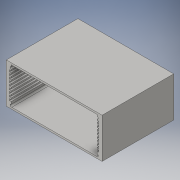
# Autodesk Inventor part: 40mm_Case
Saved by Autodesk Inventor 2016 (Build 200138000, 138)
## iProperties
Created: 2016-09-07
Part Number: 40mm_Case
Material: Generic
Document SubType Name: Modeling
Designer: jfixelle
Density: 1 g/cm^3
Appearance: Default
Author: jfixelle
Autodesk Inventor part; units mm, degrees
ref_plane "YZ Plane" through (0, 0, 0) normal (1, 0, 0) x (0, 1, 0)
ref_plane "XZ Plane" through (0, 0, 0) normal (0, 1, 0) x (-1, 0, 0)
ref_plane "XY Plane" through (0, 0, 0) normal (0, 0, 1) x (1, 0, 0)
sketch "Sketch2" plane through (0, 0, 0) normal (0, 0, 1) x (1, 0, 0)
  line L0 (-53.825, 22.5) -> (53.825, 22.5)
  line L1 (53.825, 22.5) -> (53.825, -22.5)
  line L2 (53.825, -22.5) -> (-53.825, -22.5)
  line L3 (-53.825, -22.5) -> (-53.825, 22.5)
  line L4 (-48.25, 20.5) -> (48.25, 20.5)
  line L5 (48.25, -20.5) -> (-48.25, -20.5)
  line L6 (-50.25, 19.8997) -> (-50.25, -18.4997)
  line L7 (50.25, 19.3484) -> (50.25, -18.4997)
  line L8 (48.25, 14.7) -> (50.25, 14.7)
  line L9 (-50.25, 14.7) -> (-48.25, 14.7)
  line L10 (-50.25, -15.3) -> (-48.25, -15.3)
  line L11 (48.25, -15.3) -> (50.25, -15.3)
  line L12 (49.25, 14.7) -> (49.25, -15.3) construction
  line L13 (49.25, -0.3) -> (-49.8494, -0.3) construction
  line L14 (48.25, -1.3) -> (50.25, -1.3)
  line L15 (50.25, 0.7) -> (48.25, 0.7)
  line L16 (-48.25, 0.7) -> (-50.25, 0.7)
  line L17 (-48.25, -1.3) -> (-50.25, -1.3)
  line L18 (-50.25, 2.2) -> (-48.25, 2.2)
  line L19 (48.25, 2.2) -> (50.25, 2.2)
  line L20 (-50.25, -2.8) -> (-48.25, -2.8)
  line L21 (48.25, -2.8) -> (50.25, -2.8)
  line L22 (-48.25, 4.2) -> (-50.25, 4.2)
  line L23 (48.25, 4.2) -> (50.25, 4.2)
  line L24 (50.25, -4.8) -> (48.25, -4.8)
  line L25 (-48.25, -4.8) -> (-50.25, -4.8)
  line L26 (48.25, -1.3) -> (48.25, -2.8)
  line L27 (48.25, 2.2) -> (48.25, 0.7)
  line L28 (-48.25, -2.8) -> (-48.25, -1.3)
  line L29 (-48.25, 0.7) -> (-48.25, 2.2)
  line L30 (-48.25, -6.3) -> (-50.25, -6.3)
  line L31 (48.25, -6.3) -> (50.25, -6.3)
  line L32 (48.25, -8.3) -> (50.25, -8.3)
  line L33 (-48.25, -8.3) -> (-50.25, -8.3)
  line L34 (-50.25, -9.8) -> (-48.25, -9.8)
  line L35 (48.25, -9.8) -> (50.25, -9.8)
  line L36 (50.25, -11.8) -> (48.25, -11.8)
  line L37 (-48.25, -11.8) -> (-50.25, -11.8)
  line L38 (-50.25, -13.3) -> (-48.25, -13.3)
  line L39 (48.25, -13.3) -> (50.25, -13.3)
  line L40 (50.25, 5.7) -> (48.25, 5.7)
  line L41 (-48.25, 5.7) -> (-50.25, 5.7)
  line L42 (-50.25, 7.7) -> (-48.25, 7.7)
  line L43 (48.25, 7.7) -> (50.25, 7.7)
  line L44 (50.25, 9.2) -> (48.25, 9.2)
  line L45 (-48.25, 9.2) -> (-50.25, 9.2)
  line L46 (-50.25, 11.2) -> (-48.25, 11.2)
  line L47 (48.25, 11.2) -> (50.25, 11.2)
  line L48 (50.25, 12.7) -> (48.25, 12.7)
  line L49 (-48.25, 12.7) -> (-50.25, 12.7)
  line L50 (48.25, -4.8) -> (48.25, -6.3)
  line L51 (48.25, -8.3) -> (48.25, -9.8)
  line L52 (48.25, -11.8) -> (48.25, -13.3)
  line L53 (48.25, -15.3) -> (48.25, -20.5)
  line L54 (48.25, 5.7) -> (48.25, 4.2)
  line L55 (48.25, 9.2) -> (48.25, 7.7)
  line L56 (48.25, 20.5) -> (48.25, 14.7)
  line L57 (48.25, 12.7) -> (48.25, 11.2)
  line L58 (-48.25, -20.5) -> (-48.25, -15.3)
  line L59 (-48.25, -13.3) -> (-48.25, -11.8)
  line L60 (-48.25, -9.8) -> (-48.25, -8.3)
  line L61 (-48.25, -6.3) -> (-48.25, -4.8)
  line L62 (-48.25, 4.2) -> (-48.25, 5.7)
  line L63 (-48.25, 7.7) -> (-48.25, 9.2)
  line L64 (-48.25, 11.2) -> (-48.25, 12.7)
  line L65 (-48.25, 14.7) -> (-48.25, 20.5)
  point P0 (0, 0)
  dimension "d0" = 107.65
  dimension "d1" = 53.825
  dimension "d2" = 45
  dimension "d3" = 22.5
  dimension "d4" = 96.5
  dimension "d6" = 20.5
  dimension "d7" = 20.5
  dimension "d8" = 50.25
  dimension "d9" = 50.25
  dimension "d10" = 5.8
  dimension "d11" = 5.2
  dimension "d12" = 2
  dimension "d13" = 1
  dimension "d14" = 5
  dimension "d15" = 2.5
  dimension "d16" = 2
  dimension "d17" = 5
  dimension "d18" = 9
  dimension "d19" = 4.5
  dimension "d20" = 12
  dimension "d21" = 6
  dimension "d22" = 16
  dimension "d23" = 8
  dimension "d24" = 19
  dimension "d25" = 9.5
  dimension "d26" = 23
  dimension "d27" = 11.5
  dimension "d28" = 26
  dimension "d29" = 13
  constraints: 128 end point, 103 parallel, 93 perpendicular, 32 point on line, 9 horizontal, 3 midpoint, 42 other
  measures "d0" distance of L0.start L0.end
  measures "d1" distance from line of point (0, 0) L1
  measures "d2" distance of L0.end L1.end
  measures "d3" distance from line of point (0, 0) L0
  measures "d4" distance of L4.start L4.end
  measures "d6" distance from line of point (0, 0) L4
  measures "d7" distance from line of L5 point (0, 0)
  measures "d10" distance between parallel lines of L4 L9
  measures "d11" distance between parallel lines of L5 L11
  measures "d12" distance between parallel lines of L17 L16
  measures "d13" distance between parallel lines of L17 L13
  measures "d14" distance between parallel lines of L21 L19
  measures "d15" distance between parallel lines of L13 L21
  measures "d16" distance between parallel lines of L14 L15
  measures "d17" distance between parallel lines of L20 L18
  measures "d18" distance between parallel lines of L25 L22
  measures "d19" distance between parallel lines of L13 L22
  measures "d20" distance between parallel lines of L41 L30
  measures "d21" distance between parallel lines of L13 L41
  measures "d22" distance between parallel lines of L33 L42
  measures "d23" distance between parallel lines of L13 L33
  measures "d24" distance between parallel lines of L45 L34
  measures "d25" distance between parallel lines of L13 L34
  measures "d26" distance between parallel lines of L46 L37
  measures "d27" distance between parallel lines of L13 L46
  measures "d28" distance between parallel lines of L49 L38
  measures "d29" distance between parallel lines of L13 L49
extrude "Extrusion1" add sketch "Sketch2" along normal blind 80.5 contours L0 L1 L2 L3 | L49 L64 L46 L6 | L7 L47 L57 L48 | L45 L63 L42 L6 | L7 L43 L55 L44 | L41 L62 L22 L6 | L7 L23 L54 L40 | L18 L29 L16 L6 | L7 L15 L27 L19 | L17 L28 L20 L6 | L7 L21 L26 L14 | L25 L61 L30 L6 | L7 L31 L50 L24 | L33 L60 L34 L6 | L7 L35 L51 L32 | L37 L59 L38 L6 | L7 L39 L52 L36
sketch "Sketch3" plane through (0, 0, 80.5) normal (0, 0, 1) x (1, 0, 0)
  circle A0 centre (48.25, -19.2) radius 1.4223
  circle A1 centre (48.25, 17.3) radius 1.3597
  point P0 (0, 0)
  dimension "d32" = 19.2
  dimension "d33" = 17.3
  dimension "d34" = 48.25
  dimension "d35" = 48.25
  constraints: 2 centre point
  measures "d32" vertical distance of A0.centre point (0, 0)
  measures "d33" vertical distance of A1.centre point (0, 0)
  measures "d34" horizontal distance of point (0, 0) A1.centre
  measures "d35" horizontal distance of point (0, 0) A0.centre
extrude "Extrusion2" cut sketch "Sketch3" against normal through all
mirror "Mirror1" about plane through (0, 0, 0) normal (1, 0, 0) of "Extrusion2"
body "Solid1"
